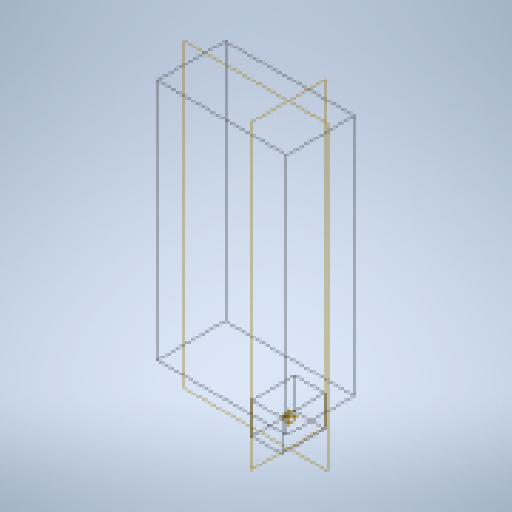
# Autodesk Inventor part: UpperArmActuatorBaseBoundingBox
Saved by Autodesk Inventor 2023 (Build 270158000, 158)
## iProperties
Created: 2023-03-24
Part Number: UpperArmActuatorBaseBoundingBox
Material: Generic
Document SubType Name: Modeling
Designer: Val
Density: 1 g/cm^3
Appearance: Default
Author: Val
Autodesk Inventor part; units mm, degrees
ref_plane "XZ Plane" through (0, 0, 0) normal (0, 1, 0) x (-1, 0, 0)
sketch "Sketch1" plane through (0, 0, 0) normal (0, 0, 1) x (1, 0, 0)
  circle A0 centre (0, 0) radius 3.175 projected
  line L0 (5.0349, -7.366) -> (-5.0349, -7.366) projected
  line L1 (-8.89, 10.922) -> (-8.89, -7.366) projected
  line L2 (8.89, -7.366) -> (8.89, 10.922) projected
  line L3 (-37.211, 10.922) -> (12.7, 10.922) construction
  line L4 (-8.89, 10.922) -> (8.89, 10.922)
  line L5 (8.89, 10.922) -> (8.89, -7.366)
  line L6 (8.89, -7.366) -> (-8.89, -7.366)
  line L7 (-8.89, -7.366) -> (-8.89, 10.922)
  constraints: 8 end point, 4 collinear, 2 parallel, 1 horizontal, 1 perpendicular
extrude "Extrusion1" add sketch "Sketch1" along normal mid plane 25.4 contours A0 | L0 L6 L1 L4 L2
ref_plane "Work Plane1" through (15.0814, 10.922, 0) normal (0, -1, 0) x (0, 0, -1)
sketch "Sketch3" plane through (15.0814, 10.922, 0) normal (0, -1, 0) x (0, 0, -1)
  line L0 (-19.939, 3.9686) -> (19.939, 3.9686)
  line L1 (19.939, 3.9686) -> (19.939, -72.2314)
  line L2 (19.939, -72.2314) -> (-19.939, -72.2314)
  line L3 (-19.939, -72.2314) -> (-19.939, 3.9686)
  line L4 (-9.525, 3.9686) -> (9.525, 3.9686) construction
  arc A0 (-19.939, -52.2924) -> (19.939, -52.2924) centre (0, -52.2924) ccw construction
  point P0 (0, -15.0814)
  point P1 (-19.939, -2.3814)
  point P2 (19.939, -2.3814)
  constraints: 8 end point, 2 parallel, 2 point on line, 1 collinear, 1 horizontal, 1 perpendicular, 1 tangent, 2 other
extrude "Extrusion2" add sketch "Sketch3" against normal blind 142.705
body "Solid1"
